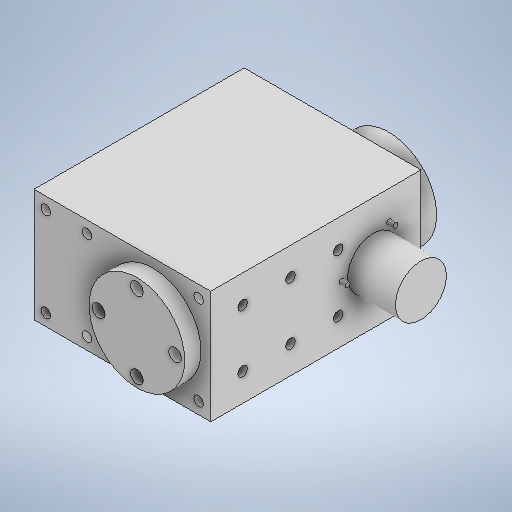
# Autodesk Inventor part: Servo_moteur_rovmaker
Saved by Autodesk Inventor 2025.1 (Build 291241000, 241)
## iProperties
Created: 2025-05-12
Part Number: Servo_moteur_rovmaker
Material: Générique
Document SubType Name: Modeling
Designer: chapuzet
Density: 1 g/cm^3
Appearance: Par défaut
Author: chapuzet
Autodesk Inventor part; units mm, degrees
ref_plane "YZ Plane" through (0, 0, 0) normal (1, 0, 0) x (0, 1, 0)
ref_plane "XZ Plane" through (0, 0, 0) normal (0, 1, 0) x (-1, 0, 0)
ref_plane "XY Plane" through (0, 0, 0) normal (0, 0, 1) x (1, 0, 0)
sketch "Esquisse1" plane through (0, 0, 0) normal (0, 1, 0) x (-1, 0, 0)
  line L0 (-27.75, 33) -> (27.75, 33)
  line L1 (27.75, 33) -> (27.75, -33)
  line L2 (27.75, -33) -> (-27.75, -33)
  line L3 (-27.75, -33) -> (-27.75, 33)
  line L4 (-27.75, 33) -> (27.75, -33) construction
  line L5 (27.75, 33) -> (-27.75, -33) construction
  point P0 (0, 0)
  dimension "d0" = 66
  dimension "d1" = 55.5
  constraints: 12 end point, 2 midpoint, 2 parallel, 1 horizontal, 1 perpendicular
  measures "d0" distance of L2.end L0.start
  measures "d1" distance of L1.end L2.end
extrude "Extrusion1" add sketch "Esquisse1" along normal blind 35.5
sketch "Esquisse2" plane through (27.75, 0, 33) normal (1, 0, 0) x (0, 0, -1)
  circle A0 centre (40, 26.75) radius 1.5
  circle A1 centre (40, 8.75) radius 1.5
  line L0 (66, 0) -> (66, 35.5) projected
  circle A2 centre (25, 8.75) radius 1.5
  circle A3 centre (25, 26.75) radius 1.5
  circle A4 centre (10, 8.75) radius 1.5
  circle A5 centre (10, 26.75) radius 1.5
  line L1 (66, 0) -> (0, 0) projected
  line L2 (40, 8.75) -> (40, 26.75)
  line L3 (40, 26.75) -> (25, 26.75)
  line L4 (25, 26.75) -> (10, 26.75)
  line L5 (10, 26.75) -> (10, 8.75)
  line L6 (10, 8.75) -> (25, 8.75)
  line L7 (25, 8.75) -> (25, 26.75)
  line L8 (25, 8.75) -> (40, 8.75)
  line L9 (40, 26.75) -> (66, 26.75)
  line L10 (40, 8.75) -> (66, 8.75)
  circle A6 centre (51, 17.75) radius 8
  circle A7 centre (41, 17.75) radius 0.75
  line L11 (0, 0) -> (0, 35.5) projected
  line L12 (0, 17.75) -> (66, 17.75)
  circle A8 centre (56, 9.0897) radius 0.75
  circle A9 centre (56, 26.4103) radius 0.75
  point P0 (33, 0)
  point P1 (40, 17.75)
  point P2 (10, 17.75)
  dimension "d4" = 18
  dimension "d5" = 3
  dimension "d22" = 16
  dimension "d27" = 1.5
  dimension "d61" = 10
  dimension "d62" = 15
  dimension "d63" = 15
  dimension "d64" = 51
  dimension "d65" = 10
  dimension "d68" = 360
  constraints: 20 end point, 10 centre point, 5 equal radius, 5 perpendicular, 5 point on line, 4 midpoint, 3 parallel, 1 collinear, 7 other
  measures "d4" distance of L2.start L2.end
  measures "d5" diameter of A0
  measures "d22" diameter of A6
  measures "d27" diameter of A7
  measures "d61" distance between parallel lines of L11 L5
  measures "d62" distance between parallel lines of L7 L5
  measures "d63" distance between parallel lines of L2 L7
  measures "d64" distance from line of L11 A6.centre
  measures "d65" distance of A6.centre A7.centre
hole "Perçage1" at (27.75, 26.75, 23) at (27.75, 26.75, 8) at (27.75, 26.75, -7) at (27.75, 8.75, -7) at (27.75, 8.75, 8) at (27.75, 8.75, 23) direction (-1, 0, 0) diameter 3 depth 5 tip angle 118
mirror "Mise en miroir1" about plane through (0, 0, 0) normal (1, 0, 0) of "Perçage1"
extrude "Extrusion2" add sketch "Esquisse2" along normal blind 2 contours A9 L9 | L9 A9 | L12 A7 | A7 L12 | A8 L10 | L10 A8
extrude "Extrusion3" add sketch "Esquisse2" along normal blind 15 contours L12 A6 | A6 L12
sketch "Esquisse4" plane through (-27.75, 0, 33) normal (0, 0, 1) x (1, 0, 0)
  circle A0 centre (37.4, 17.75) radius 15
  line L0 (0, 0) -> (55.5, 0) projected
  circle A1 centre (51.7, 31.75) radius 1.5
  circle A2 centre (51.7, 3.75) radius 1.5
  line L1 (55.5, 0) -> (55.5, 35.5) projected
  line L2 (55.5, 3.75) -> (51.7, 3.75)
  line L3 (51.7, 3.75) -> (51.7, 31.75)
  line L4 (51.7, 31.75) -> (55.5, 31.75)
  circle A3 centre (16.7, 31.75) radius 1.5
  circle A4 centre (16.7, 3.75) radius 1.5
  circle A5 centre (3.7, 31.75) radius 1.5
  circle A6 centre (3.7, 3.75) radius 1.5
  line L5 (16.7, 31.75) -> (16.7, 3.75)
  line L6 (16.7, 3.75) -> (3.7, 3.75)
  line L7 (3.7, 3.75) -> (3.7, 31.75)
  line L8 (3.7, 31.75) -> (16.7, 31.75)
  line L9 (51.7, 31.75) -> (16.7, 31.75)
  line L10 (16.7, 3.75) -> (51.7, 3.75)
  circle A7 centre (37.4, 5.75) radius 2
  circle A8 centre (37.4, 17.75) radius 12
  circle A9 centre (49.4, 17.75) radius 2
  circle A10 centre (37.4, 29.75) radius 2
  circle A11 centre (25.4, 17.75) radius 2
  line L11 (0, 0) -> (0, 35.5) projected
  point P0 (27.75, 0)
  point P1 (51.7, 17.75)
  dimension "d40" = 24
  dimension "d32" = 17.75
  dimension "d33" = 30
  dimension "d34" = 28
  dimension "d35" = 3
  dimension "d36" = 3.8
  dimension "d38" = 35
  dimension "d39" = 13
  dimension "d41" = 4
  dimension "d44" = 360
  dimension "d48" = 17.75
  dimension "d59" = 37.4
  dimension "d60" = 18.1
  dimension "d70" = 3.7
  constraints: 18 end point, 11 centre point, 5 equal radius, 4 perpendicular, 2 parallel, 2 point on line, 1 coincident, 1 collinear, 1 horizontal, 1 midpoint, 1 vertical, 1 vertical alignment, 11 other
  measures "d32" distance from line of L0 A0.centre
  measures "d33" diameter of A0
  measures "d34" distance of L3.end L2.end
  measures "d35" diameter of A2
  measures "d36" distance from line of L1 L2.end
  measures "d38" distance of L5.end L2.end
  measures "d39" distance of L5.end L6.end
  measures "d41" diameter of A7
  measures "d48" distance from line of L0 point (51.7, 17.75)
  measures "d59" distance from line of L11 point (37.4, 17.75)
  measures "d60" distance from line of L1 A0.centre
  measures "d70" distance from line of L11 L6.end
extrude "Extrusion4" add sketch "Esquisse4" along normal blind 5.1 contours A0 L3 | L3 A0 L10 A7 A8 A9 A10 L9 | L9 A0 | A0 L10 | L9 A10 A8 A11 A7 L10 A0 | A10 A8 A9 A7 A11
hole "Perçage2" at (23.95, 31.75, 33) at (23.95, 3.75, 33) at (-11.05, 3.75, 33) at (-24.05, 3.75, 33) at (-24.05, 31.75, 33) at (-11.05, 31.75, 33) direction (0, 0, -1) diameter 3 depth 6 tip angle 118
sketch "Esquisse5" plane through (27.75, 0, -33) normal (0, 0, -1) x (-1, 0, 0)
  circle A0 centre (18.1, 17.75) radius 15 projected
  circle A1 centre (18.1, 17.75) radius 15
  circle A2 centre (6.1, 17.75) radius 2 projected
  circle A3 centre (6.1, 17.75) radius 2
  circle A4 centre (18.1, 29.75) radius 2 projected
  circle A5 centre (18.1, 29.75) radius 2
  circle A6 centre (30.1, 17.75) radius 2 projected
  circle A7 centre (30.1, 17.75) radius 2
  circle A8 centre (18.1, 5.75) radius 2 projected
  circle A9 centre (18.1, 5.75) radius 2
  point P0 (27.75, 0)
  dimension "d56" = 30
  constraints: 5 centre point, 5 coincident
  measures "d56" diameter of A0
extrude "Extrusion5" add sketch "Esquisse5" along normal blind 8
